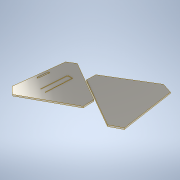
# Autodesk Inventor part: Bottom
Saved by Autodesk Inventor 2020.2 (Build 242310000, 310)
## iProperties
Created: 2021-02-25
Part Number: Bottom
Material: Titanium
Document SubType Name: Modeling
Designer: saika
Density: 4.51 g/cm^3
Appearance: Titanium
Author: saika
Autodesk Inventor part; units mm, degrees
ref_plane "YZ Plane" through (0, 0, 0) normal (1, 0, 0) x (0, 1, 0)
ref_plane "XZ Plane" through (0, 0, 0) normal (0, 1, 0) x (-1, 0, 0)
ref_plane "XY Plane" through (0, 0, 0) normal (0, 0, 1) x (1, 0, 0)
sketch "Sketch1" plane through (0, 0, 0) normal (0, 1, 0) x (-1, 0, 0)
  line L0 (25.0398, -0.2818) -> (28.6005, -0.2818)
  line L1 (29.7875, 0.9051) -> (29.7875, 29.3913)
  line L2 (23.8528, 29.3913) -> (23.8528, 0.9051)
  arc A0 (28.6005, -0.2818) -> (29.7875, 0.9051) centre (28.6005, 0.9051) ccw
  arc A1 (23.8528, 0.9051) -> (25.0398, -0.2818) centre (25.0398, 0.9051) ccw
  line L3 (24.4463, -0.8753) -> (29.194, -0.8753)
  line L4 (30.3809, 0.3117) -> (30.3809, 29.3913)
  line L5 (23.2594, 29.3913) -> (23.2594, 0.3117)
  arc A2 (29.194, -0.8753) -> (30.3809, 0.3117) centre (29.194, 0.3117) ccw
  arc A3 (23.2594, 0.3117) -> (24.4463, -0.8753) centre (24.4463, 0.3117) ccw
  line L6 (29.7875, 29.3913) -> (30.3809, 29.3913)
  line L7 (23.8528, 29.3913) -> (23.2594, 29.3913)
  line L8 (-11.8158, 20.3083) -> (40.1457, 50.3083)
  line L9 (-11.8158, 8.3083) -> (40.1457, -21.6917)
  line L10 (50.538, 44.3083) -> (50.538, -15.6917)
  line L11 (50.538, 44.3083) -> (40.1457, 50.3083)
  line L12 (50.538, -15.6917) -> (40.1457, -21.6917)
  line L13 (-11.8158, 20.3083) -> (-11.8158, 8.3083)
  line L14 (-39.0112, 22.4219) -> (12.9503, -7.5781)
  line L15 (-49.4035, 16.4219) -> (-49.4035, -43.5781)
  line L16 (12.9503, -19.5781) -> (-39.0112, -49.5781)
  line L17 (12.9503, -19.5781) -> (12.9503, -7.5781)
  line L18 (-39.0112, -49.5781) -> (-49.4035, -43.5781)
  line L19 (-39.0112, 22.4219) -> (-49.4035, 16.4219)
  line L20 (45.3419, 20.3083) -> (45.3419, 8.3083)
  line L21 (47.3419, 8.3083) -> (47.3419, 20.3083)
  arc A4 (47.3419, 20.3083) -> (45.3419, 20.3083) centre (46.3419, 20.3083) ccw
  arc A5 (45.3419, 8.3083) -> (47.3419, 8.3083) centre (46.3419, 8.3083) ccw
  point P0 (0, 0)
  point P1 (0.0037, 0.0061)
  constraints: 44 end point, 12 point on circle, 12 tangent, 6 centre point, 4 perpendicular, 2 horizontal, 2 parallel, 1 equal radius, 1 vertical
extrude "Extrusion1" add sketch "Sketch1" along normal blind 1.6
body "Solid1"
